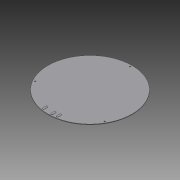
# Autodesk Inventor part: Heatbed_Geeetech_215mm
Saved by Autodesk Inventor 2014 (Build 180170000, 170)
## iProperties
Created: 2015-02-09
Part Number: Heatbed_Geeetech_215mm
Material: Generic
Document SubType Name: Modeling
Designer: ThatOtherGuy
Density: 1 g/cm^3
Appearance: Default
Author: ThatOtherGuy
Autodesk Inventor part; units mm, degrees
ref_plane "YZ Plane" through (0, 0, 0) normal (1, 0, 0) x (0, 1, 0)
ref_plane "XZ Plane" through (0, 0, 0) normal (0, 1, 0) x (-1, 0, 0)
ref_plane "XY Plane" through (0, 0, 0) normal (0, 0, 1) x (1, 0, 0)
sketch "Sketch1" plane through (0, 0, 0) normal (0, 0, 1) x (1, 0, 0)
  circle A0 centre (0, 0) radius 107.5
  dimension "d0" = 215
  constraints: 1 centre point, 1 coincident
  measures "d0" diameter of A0
extrude "Extrusion1" add sketch "Sketch1" along normal blind 1.6
sketch "Sketch2" plane through (0, 0, 1.6) normal (0, 0, 1) x (1, 0, 0)
  circle A0 centre (0, 0) radius 107.5 projected
  line L0 (0, 102.5) -> (0, 0) construction
  dimension "d3" = 102.5
  constraints: 2 end point, 1 vertical
  measures "d3" distance of L0.start L0.end
hole "Hole1" at (0, 102.5, 1.6) direction (0, 0, -1) diameter 3 end through all
pattern_circular "Circular Pattern1" count 3 over 360 about axis through (0, 0, 0) along (0, 0, 1) of "Hole1"
sketch "Sketch3" plane through (0, 0, 1.6) normal (0, 0, 1) x (1, 0, 0)
  circle A0 centre (0, 0) radius 107.5 projected
  line L0 (-17.5, -93.495) -> (-17.5, -100.995) construction
  line L1 (-20, -93.495) -> (-20, -100.995)
  line L2 (-15, -100.995) -> (-15, -93.495)
  arc A1 (-15, -93.495) -> (-20, -93.495) centre (-17.5, -93.495) ccw
  arc A2 (-20, -100.995) -> (-15, -100.995) centre (-17.5, -100.995) ccw
  line L3 (5, -94.9305) -> (5, -102.4305) construction
  line L4 (2.5, -94.9305) -> (2.5, -102.4305)
  line L5 (7.5, -102.4305) -> (7.5, -94.9305)
  arc A3 (7.5, -94.9305) -> (2.5, -94.9305) centre (5, -94.9305) ccw
  arc A4 (2.5, -102.4305) -> (7.5, -102.4305) centre (5, -102.4305) ccw
  line L6 (17.5, -93.495) -> (17.5, -100.995) construction
  line L7 (15, -93.495) -> (15, -100.995)
  line L8 (20, -100.995) -> (20, -93.495)
  arc A5 (20, -93.495) -> (15, -93.495) centre (17.5, -93.495) ccw
  arc A6 (15, -100.995) -> (20, -100.995) centre (17.5, -100.995) ccw
  arc A7 (-17.5, -97.245) -> (17.5, -97.245) centre (0, 0) ccw construction
  line L9 (-17.5, -97.245) -> (17.5, -97.245) construction
  point P0 (5, -98.6805)
  dimension "d14" = 7.5
  dimension "d15" = 2.5
  dimension "d16" = 35
  dimension "d17" = 2.5
  dimension "d18" = 12.5
  constraints: 26 end point, 15 point on circle, 12 tangent, 7 centre point, 7 parallel, 3 midpoint, 2 equal radius, 1 concentric, 1 horizontal, 1 vertical
  measures "d14" distance of L0.start L0.end
  measures "d15" radius of A1
  measures "d16" distance of L9.start L9.end
  measures "d18" distance between parallel lines of L6 L3
extrude "Extrusion2" add sketch "Sketch3" along normal blind 0.5 draft -10 contours A1 L2 A2 L1 | A3 L5 A4 L4 | A5 L8 A6 L7
body "Solid1"
